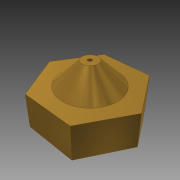
# Autodesk Inventor part: nozzle
Saved by Autodesk Inventor 2014 (Build 180170000, 170)
## iProperties
Created: 2014-03-25
Part Number: nozzle
Material: Brass, Soft Yellow
Document SubType Name: Modeling
Designer: buben
Density: 8.47 g/cm^3
Appearance: Brass - Satin
Mass: 1.58376 g
Surface Area: 2.09131 cm^2
Volume: 0.186985 cm^3
Author: buben
Autodesk Inventor part; units mm, degrees
ref_plane "XZ Plane" through (0, 0, 0) normal (0, 1, 0) x (-1, 0, 0)
ref_plane "XY Plane" through (0, 0, 0) normal (0, 0, 1) x (1, 0, 0)
sketch "Sketch1" plane through (0, 0, 0) normal (0, 0, 1) x (1, 0, 0)
  line L0 (2.3094, 4) -> (4.6188, 0)
  line L1 (4.6188, 0) -> (2.3094, -4)
  line L2 (2.3094, -4) -> (-2.3094, -4)
  line L3 (-2.3094, -4) -> (-4.6188, 0)
  line L4 (-4.6188, 0) -> (-2.3094, 4)
  line L5 (-2.3094, 4) -> (2.3094, 4)
  point P0 (0, 0)
  point P1 (0, 0)
  dimension "d0" = 8
  constraints: 12 end point, 1 coincident, 1 horizontal, 13 other
  measures "d0" distance between parallel lines of L2 L5
extrude "Extrusion1" add sketch "Sketch1" along normal blind 3
ref_plane "Work Plane1" through (0, 0, 0) normal (1, 0, 0) x (0, 1, 0)
sketch "Sketch2" plane through (0, 0, 0) normal (1, 0, 0) x (0, 1, 0)
  line L0 (0, 0) -> (-4, 0) projected
  line L1 (0, 0) -> (0, 3) projected
  line L2 (-4, 3) -> (0, 3) projected
  line L3 (-4, 0) -> (-4, 3) projected
  line L4 (4, 0) -> (0, 0) projected
  line L5 (4, 0) -> (4, 3) projected
  line L6 (0, 3) -> (4, 3) projected
  line L7 (0, 0) -> (0, 3) projected
  line L8 (0, 3) -> (0, 5)
  line L9 (0, 5) -> (0.75, 5)
  line L10 (0.75, 5) -> (2.75, 3)
  line L11 (0, 3) -> (2.75, 3)
  point P0 (0, 0)
  dimension "d4" = 2
  dimension "d5" = 0.75
  dimension "d6" = 2.75
  constraints: 8 end point, 2 parallel, 1 collinear, 1 point on line
  measures "d4" distance of L6.start L8.end
  measures "d5" distance of L8.end L9.end
  measures "d6" distance of L1.end L10.end
revolve "Revolution1" add sketch "Sketch2" angle 360 about axis through (0, 0, 3) along (0, 0, 1) contours L8 L9 L10 L6
sketch "Sketch3" plane through (0, 0, 5) normal (0, 0, 1) x (1, 0, 0)
  circle A0 centre (0, 0) radius 0.75 projected
  circle A1 centre (0, 0) radius 0.2
  dimension "d8" = 0.4
  constraints: 1 centre point, 1 coincident
  measures "d8" diameter of A1
extrude "Extrusion2" cut sketch "Sketch3" against normal through all contours A1
body "Solid1"
